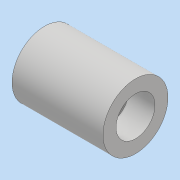
# Autodesk Inventor part: P2
Saved by Autodesk Inventor 2017 (Build 210142000, 142)
## iProperties
Part Number: P2
Material: 一般
Document SubType Name: Modeling
Designer: d8910
Density: 1 g/cm^3
Appearance: 預設
Author: d8910
Autodesk Inventor part; units mm, degrees
ref_plane "YZ Plane" through (0, 0, 0) normal (1, 0, 0) x (0, 1, 0)
ref_plane "XZ Plane" through (0, 0, 0) normal (0, 1, 0) x (-1, 0, 0)
ref_plane "XY Plane" through (0, 0, 0) normal (0, 0, 1) x (1, 0, 0)
sketch "草圖1" plane through (0, 0, 0) normal (0, 0, 1) x (1, 0, 0)
  line L0 (-70, 0) -> (70, 0)
  line L1 (70, 0) -> (70, 50)
  line L2 (70, 50) -> (-70, 50)
  line L3 (-70, 50) -> (-70, 0)
  line L4 (-50, 0) -> (30, 0)
  line L5 (30, 0) -> (30, 10)
  line L6 (30, 10) -> (-50, 10)
  line L7 (-50, 10) -> (-50, 0)
  line L8 (30, 0) -> (70, 0)
  line L9 (70, 0) -> (70, 30)
  line L10 (70, 30) -> (30, 30)
  line L11 (30, 30) -> (30, 0)
  point P0 (0, 0)
  point P1 (0, 50)
  dimension "d0" = 140
  dimension "d1" = 50
  dimension "d2" = 40
  dimension "d3" = 120
  dimension "d4" = 30
  dimension "d5" = 10
  constraints: 24 end point, 6 parallel, 3 horizontal, 3 perpendicular, 2 point on line, 1 horizontal alignment, 1 midpoint, 1 vertical alignment
  measures "d0" distance of L1.end L2.end
  measures "d1" distance of L0.end L1.end
  measures "d2" distance of L9.end L10.end
  measures "d3" distance between parallel lines of L1 L7
  measures "d4" distance between parallel lines of L0 L10
  measures "d5" distance between parallel lines of L0 L6
revolve "迴轉1" add sketch "草圖1" angle 360 about axis through (-50, 0, 0) along (1, 0, 0) contours L3 L2 L1 L10 L11 L6 L7 L0
